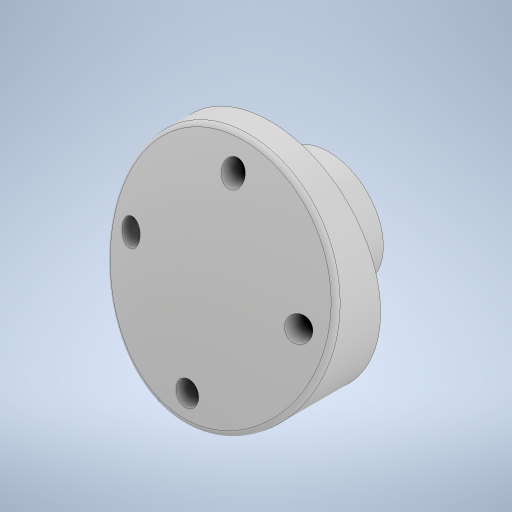
# Autodesk Inventor part: 메인 형상_상단
Saved by Autodesk Inventor 2023 (Build 270158000, 158)
## iProperties
Created: 2022-06-06
Part Number: 메인 형상_상단
Material: 일반
Document SubType Name: Modeling
Designer: fly01
Density: 1 g/cm^3
Appearance: 기본값
Author: fly01
Autodesk Inventor part; units mm, degrees
sketch "스케치1" plane through (0, 0, 0) normal (0, 0, 1) x (1, 0, 0)
  line L0 (-71.7255, 0) -> (71.7255, 0)
  circle A0 centre (0, 90) radius 60
  line L1 (0, 90) -> (0, 0)
  circle A1 centre (0, 30.8371) radius 28.5 construction
  line L2 (-71.7255, 0) -> (-71.7255, 37.2069) construction
  line L3 (-71.7255, 37.2069) -> (-78.5321, 115.9482) construction
  line L4 (-78.5321, 115.9482) -> (-27.826, 143.1575) construction
  spline S0 degree 3 poles (-71.7255, 0) (-71.7255, 37.2069) (-78.5321, 115.9482) (-27.826, 143.1575) knots 1 1 1 1 2 2 2 2
  line L5 (0, 90) -> (0, 150)
  arc A2 (0, 145) -> (-25.4845, 138.7395) centre (0, 90) ccw
  line L6 (0, 30) -> (-67.0278, 30)
  circle A3 centre (0, 90) radius 3.75
  spline S1 degree 5 poles (-66.7255, 0) (-66.7263, 5.3162) (-66.8357, 10.6319) (-66.9373, 15.9467) (-67.1005, 27.5918) (-66.983, 39.2375) (-66.7938, 45.566) (-66.085, 58.4226) (-64.543, 71.2073) (-63.4967, 77.671) (-60.8372, 90.1616) (-56.6655, 102.2287) (-54.2155, 107.9557) (-48.3515, 118.8219) (-40.3438, 128.214) (-35.8227, 132.3719) (-30.8109, 135.8802) (-25.4618, 138.7517) knots 0 0 0 0 0 0 0.174516 0.174516 0.174516 0.382289 0.382289 0.382289 0.597001 0.597001 0.597001 0.800678 0.800678 0.800678 1 1 1 1 1 1
  dimension "d6" = 5
  dimension "d0" = 143.451
  dimension "d1" = 120
  dimension "d2" = 90
  dimension "d3" = 57
  dimension "d5" = 5
  dimension "d76" = 7.5
  constraints: 8 end point, 5 point on circle, 4 centre point, 4 point on line, 2 coincident, 2 vertical, 1 horizontal, 1 midpoint, 1 perpendicular, 1 tangent, 8 other
  measures "d0" distance of L0.start L0.end
  measures "d1" diameter of A0
  measures "d2" distance of L1.start L1.end
  measures "d3" diameter of A1
  measures "d5" radial gap between concentric circles of A0 A2
  measures "d76" diameter of A3
revolve "회전1" add sketch "스케치1" angle 360 about axis through (0, 90, 0) along (0, -1, 0) picked at (-2.4818, 90) contours S0 A0 S1 L0 | S0 A0 L5 A2 S1 | A0 S0 | S1 A0 L6 | S1 A2 L5 A3 L1 A0 | A3 L5 L1
ref_plane "작업 평면3" through (0, 90, 0) normal (0, -1, 0) x (1, 0, 0)
sketch "스케치19" plane through (0, 90, 0) normal (0, -1, 0) x (1, 0, 0)
  circle A0 centre (0, 0) radius 60.5
  line L0 (98.4693, -50) -> (-98.4693, -50)
  line L1 (-98.4693, -50) -> (-98.4693, 50)
  line L2 (-98.4693, 50) -> (98.4693, 50)
  line L3 (98.4693, 50) -> (98.4693, -50)
  line L4 (98.4693, -50) -> (-98.4693, 50) construction
  line L5 (-98.4693, -50) -> (98.4693, 50) construction
  line L6 (0, -50) -> (0, 50)
  point P0 (34.0624, -50)
  point P1 (34.0624, 50)
  dimension "d73" = 121
  dimension "d74" = 100
  constraints: 14 end point, 4 midpoint, 2 parallel, 1 centre point, 1 coincident, 1 horizontal, 1 perpendicular
  measures "d73" diameter of A0
  measures "d74" distance of L2.end L0.start
revolve "회전4" cut sketch "스케치19" angle 360 about axis through (0, 90, -50) along (0, 0, 1) picked at (20.1667, 0) contours A0 L0 L6 L2
fillet "모깎기5" radius 2 1 edges at (50.5199, 123.2865, -0.0031)
sketch "스케치24" plane through (0, 30, 0) normal (0, -1, 0) x (1, 0, 0)
  circle A0 centre (0, 0) radius 67.0278
  constraints: 1 centre point, 1 coincident
extrude "돌출16" add sketch "스케치24" along normal blind 5
sketch "스케치25" plane through (0, 25, 0) normal (0, -1, 0) x (1, 0, 0)
  circle A0 centre (0, 0) radius 40
  dimension "d93" = 80
  constraints: 1 centre point, 1 coincident
  measures "d93" diameter of A0
extrude "돌출18" cut sketch "스케치25" against normal blind 154.25
ref_plane "작업 평면5" through (0, 0, 53.5) normal (0, 0, 1) x (1, 0, 0)
sketch "스케치27" plane through (0, 0, 53.5) normal (0, 0, 1) x (1, 0, 0)
  circle A0 centre (0, 90) radius 3.75
  circle A1 centre (0, 90) radius 19.75
  circle A2 centre (0, 90) radius 128.7121
  point P0 (0, 0)
  dimension "d98" = 39.5
  dimension "d109" = 7.5
  constraints: 3 centre point, 2 coincident
  measures "d98" diameter of A1
  measures "d109" diameter of A0
extrude "돌출19" cut sketch "스케치27" along normal blind 154.25 contours A2
extrude "돌출20" cut sketch "스케치27" against normal blind 154.25 contours A0 | A1 | A2
sketch "스케치28" plane through (0, 90, 53.5) normal (0, 0, -1) x (-1, 0, 0)
  circle A0 centre (0, 0) radius 9.75
  circle A1 centre (0, 0) radius 11.5
  point P0 (0, -90)
  dimension "d103" = 19.5
  dimension "d104" = 23
  constraints: 2 centre point, 1 coincident
  measures "d103" diameter of A0
  measures "d104" diameter of A1
extrude "돌출21" add sketch "스케치28" along normal blind 4
extrude "돌출22" add sketch "스케치28" along normal blind 10 contours A0
sketch "스케치29" plane through (0, 90, 53.5) normal (0, 0, -1) x (-1, 0, 0)
  circle A0 centre (0, 0) radius 19.75 projected
  circle A1 centre (0, 0) radius 11.5 projected
  point P0 (0, -90)
extrude "돌출23" cut sketch "스케치29" against normal blind 0.5
fillet "모깎기7" radius 1 2 edges at (-19.0516, 95.2055, 61.2643) (18.8155, 83.9967, 64.4226)
ref_plane "작업 평면6" through (0, 90, 57) normal (0, 0, -1) x (-1, 0, 0)
sketch "스케치30" plane through (0, 90, 57) normal (0, 0, -1) x (-1, 0, 0)
  circle A0 centre (0, 0) radius 15
  circle A1 centre (0, 15) radius 1.2
  circle A2 centre (0, 15) radius 2
  circle A3 centre (-15, 0) radius 1.2
  circle A4 centre (0, -15) radius 1.2
  circle A5 centre (15, 0) radius 1.2
  circle A6 centre (-15, 0) radius 2
  circle A7 centre (0, -15) radius 2
  circle A8 centre (15, 0) radius 2
  point P0 (0, -90)
  point P1 (-1.9956, -14.8667)
  point P2 (1.9956, -14.8667)
  point P3 (1.199, -14.952)
  point P4 (-1.199, -14.952)
  dimension "d114" = 30
  dimension "d115" = 2.4
  dimension "d116" = 4
  dimension "d119" = 360
  dimension "d123" = 360
  constraints: 8 centre point, 1 coincident, 21 other
  measures "d115" diameter of A1
  measures "d116" diameter of A2
extrude "돌출24" cut sketch "스케치30" along normal blind 7.25 contours A0 A5 | A0 A5 | A1 A0 | A0 A1 | A4 A0 | A0 A4 | A3 A0 | A0 A3
extrude "돌출25" cut sketch "스케치30" against normal blind 26.25 contours A0 A5 | A0 A5 | A5 A0 A8 | A0 A8 A5 | A2 A0 A1 | A0 A1 A2 | A7 A0 A4 | A0 A4 A7 | A1 A0 | A0 A1 | A4 A0 | A0 A4 | A6 A0 A3 | A0 A3 A6 | A3 A0 | A0 A3
sketch "스케치31" plane through (0, 90, 49.5) normal (0, 0, -1) x (-1, 0, 0)
  circle A0 centre (0, 0) radius 11.5 projected
  circle A1 centre (0, 0) radius 9.75 projected
  point P0 (0, -90)
extrude "돌출26" cut sketch "스케치31" against normal blind 0.15
